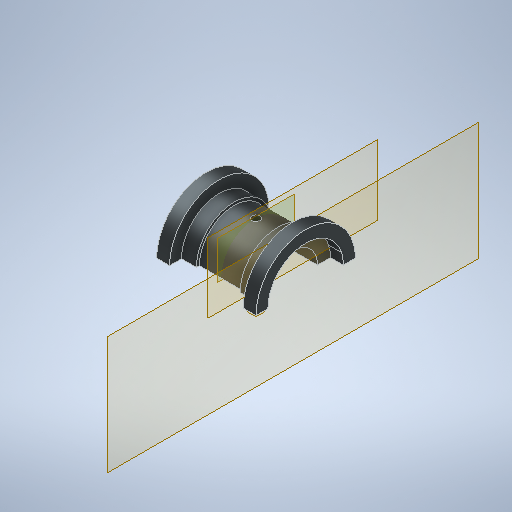
# Autodesk Inventor part: BEARING TOP
Saved by Autodesk Inventor 2025.2 (Build 292293000, 293)
## iProperties
Created: 2025-04-15
Part Number: BEARING TOP
Material: Iron, Gray
Document SubType Name: Modeling
Designer: bless
Density: 7.15 g/cm^3
Appearance: Iron Gray
Author: bless
Autodesk Inventor part; units mm, degrees
ref_plane "YZ Plane" through (0, 0, 0) normal (1, 0, 0) x (0, 1, 0)
ref_plane "XZ Plane" through (0, 0, 0) normal (0, 1, 0) x (-1, 0, 0)
ref_plane "XY Plane" through (0, 0, 0) normal (0, 0, 1) x (1, 0, 0)
ref_plane "Work Plane1" through (7.7698, -13.6706, 100.9039) normal (1, 0, 0) x (0, 1, 0)
sketch "Sketch1" plane through (7.7698, -13.6706, 100.9039) normal (1, 0, 0) x (0, 1, 0)
  arc A0 (-13, -56.8488) -> (-13, -20.7888) centre (-19.0031, -38.8188) ccw projected
  line L0 (-26, -56.8488) -> (-13, -56.8488) projected
  line L1 (-13, -20.7888) -> (-26, -20.7888) projected
  arc A1 (-19.0031, -51.3188) -> (-19.0031, -26.3188) centre (-19.0031, -38.8188) ccw
  arc A2 (-19.0031, -56.3188) -> (-19.0031, -21.3188) centre (-19.0031, -38.8188) ccw
  arc A3 (-19.0031, -63.8188) -> (-19.0031, -13.8188) centre (-19.0031, -38.8188) ccw
  line L2 (-19.0031, -13.8188) -> (-19.0031, -63.8188)
  arc A4 (-13, -56.8488) -> (-13, -20.7888) centre (-19.0031, -38.8188) ccw projected
  arc A5 (-19.0031, -57.8188) -> (-19.0031, -19.8188) centre (-19.0031, -38.8188) ccw
  point P0 (13.6706, -100.9039)
  point P1 (-13.0099, -20.7888)
  point P2 (-13.0099, -56.8488)
  dimension "d0" = 12.5
  dimension "d1" = 17.5
  dimension "d2" = 25
  dimension "d3" = 19
  constraints: 8 point on circle, 6 point on line, 4 centre point, 4 coincident, 2 end point, 1 midpoint, 1 perpendicular
  measures "d0" radius of A1
  measures "d1" radius of A2
  measures "d2" radius of A3
  measures "d3" radius of A5
extrude "Extrusion1" add sketch "Sketch1" along normal blind 6.5 contours A0 L1 A5 L2 A3 L0
ref_plane "Work Plane2" through (7.7698, -40.6706, 62.0852) normal (1, 0, 0) x (0, 1, 0)
sketch "Sketch2" plane through (7.7698, -40.6706, 62.0852) normal (1, 0, 0) x (0, 1, 0)
  arc A0 (14, -18.03) -> (14, 18.03) centre (7.9969, 0) ccw projected
  arc A1 (7.9969, -19.0031) -> (7.9969, 19.0031) centre (7.9969, 0) ccw
  arc A2 (7.9969, -17.5) -> (7.9969, 17.5) centre (7.9969, 0) ccw
  line L0 (7.9969, 19.0031) -> (7.9969, -19.0031)
  point P0 (40.6706, -62.0852)
  point P1 (14, 18.03)
  dimension "d6" = 17.5
  constraints: 4 point on circle, 2 centre point, 2 coincident, 2 end point, 2 point on line, 1 concentric, 1 midpoint, 1 vertical
  measures "d6" radius of A2
extrude "Extrusion2" add sketch "Sketch2" against normal blind 7.5 contours A1 L0 A2 A0
sketch "Sketch3" plane through (7.7698, -40.6706, 62.0852) normal (1, 0, 0) x (0, 0, -1)
  arc A0 (17.5, 7.9969) -> (-17.5, 7.9969) centre (0, 7.9969) ccw projected
  arc A1 (18.03, 14) -> (-18.03, 14) centre (0, 7.9969) ccw projected
  arc A2 (12.5, 7.9969) -> (-12.5, 7.9969) centre (0, 7.9969) ccw
  line L0 (-17.5, 7.9969) -> (17.5, 7.9969)
  point P0 (62.0852, 40.6706)
  dimension "d9" = 12.5
  constraints: 2 end point, 2 point on circle, 2 point on line, 1 centre point, 1 coincident, 1 horizontal, 1 midpoint
  measures "d9" radius of A2
extrude "Extrusion3" add sketch "Sketch3" against normal blind 18.5 contours L0 A2 A0
ref_plane "Work Plane3" through (-10.7302, -40.6706, 62.0852) normal (-1, 0, 0) x (0, 0, 1)
mirror "Mirror1" about plane through (-10.7302, -40.6706, 62.0852) normal (-1, 0, 0) of "Extrusion1", "Extrusion2", "Extrusion3"
ref_plane "Work Plane4" through (-10.7262, -56.0476, 62.0852) normal (0, 1, 0) x (-1, 0, 0)
sketch "Sketch4" plane through (-10.7262, -56.0476, 62.0852) normal (0, 1, 0) x (-1, 0, 0)
  spline S0 degree 3 poles (0, 2) (0.2512, 2) (0.5191, 1.9498) (1.0118, 1.7457) (1.2367, 1.5918) (1.5918, 1.2367) (1.7457, 1.0118) (1.9498, 0.5191) (2, 0.2512) (2, -0.2512) (1.9498, -0.5191) (1.7457, -1.0118) (1.5918, -1.2367) (1.2367, -1.5918) (1.0118, -1.7457) (0.5191, -1.9498) (0.2512, -2) (-0.2512, -2) (-0.5191, -1.9498) (-1.0118, -1.7457) (-1.2367, -1.5918) (-1.5918, -1.2367) (-1.7457, -1.0118) (-1.9498, -0.5191) (-2, -0.2512) (-2, 0.2512) (-1.9498, 0.5191) (-1.7457, 1.0118) (-1.5918, 1.2367) (-1.2367, 1.5918) (-1.0118, 1.7457) (-0.5191, 1.9498) (-0.2512, 2) (0, 2) knots 0 0 0 0 0.075352 0.075352 0.150705 0.150705 0.226057 0.226057 0.301409 0.301409 0.376761 0.376761 0.452114 0.452114 0.527466 0.527466 0.602818 0.602818 0.67817 0.67817 0.753523 0.753523 0.828875 0.828875 0.904227 0.904227 0.979579 0.979579 1.054932 1.054932 1.130284 1.130284 1.205636 1.205636 1.205636 1.205636 projected
  point P0 (-10.7262, -62.0852)
  point P1 (0, 2)
extrude "Extrusion4" cut sketch "Sketch4" along normal through all
body "Solid1"
